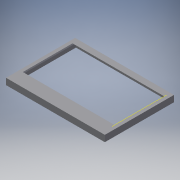
# Autodesk Inventor part: Auschnitt2
Saved by Autodesk Inventor 2017 SP1 (Build 210196100, 196)
## iProperties
Part Number: Auschnitt2
Material: Generisch
Document SubType Name: Modeling
Designer: aXe
Density: 1 g/cm^3
Appearance: Vorgabe
Author: aXe
Autodesk Inventor part; units mm, degrees
ref_plane "YZ Plane" through (0, 0, 0) normal (1, 0, 0) x (0, 1, 0)
ref_plane "Arbeitsebene1" through (47.05, -25.35, -1.6) normal (1, 0, 0) x (0, 1, 0)
sketch "Skizze1" plane through (47.05, -25.35, -1.6) normal (1, 0, 0) x (0, 1, 0)
  line L0 (0, 0) -> (50.7, 0) projected
  line L1 (50.7, 0) -> (50.7, 1.5) projected
  line L2 (0, 1.5) -> (50.7, 1.5) projected
  line L3 (0, 0) -> (0, 1.5) projected
  line L4 (-10, -1.15) -> (53.1, -1.15) projected
  line L5 (53.1, -1.15) -> (53.1, 0) projected
  line L6 (-10, 0) -> (53.1, 0) projected
  line L7 (-10, -1.15) -> (-10, 0) projected
  line L8 (0, 1.5) -> (-0.15, 1.5)
  line L9 (50.7, 1.5) -> (50.85, 1.5)
  line L10 (50.85, 1.5) -> (50.85, 1.3)
  line L11 (53.1, 0) -> (53.4, 0)
  line L12 (50.85, 1.3) -> (53.4, 0)
  line L13 (58.1558, 1.5) -> (50.85, 1.5)
  line L14 (-0.15, 1.5) -> (-0.15, 1.3)
  line L15 (-10, 0) -> (-10.3, 0)
  line L16 (-10, -1.15) -> (-18.8032, -1.15)
  line L17 (-0.15, 1.3) -> (-10.3, 0)
  line L18 (53.4, 0) -> (54.4, -1)
  line L19 (54.4, -1) -> (54.55, -1.15)
  line L20 (54.55, -1.15) -> (55.55, -1.15)
  line L21 (55.55, -1.15) -> (57.05, -1.15)
  line L22 (57.05, -1.15) -> (57.05, 1.5)
  line L23 (-10.3, 0) -> (-11.45, -1.15)
  line L24 (-11.45, -1.15) -> (-13.95, -1.15)
  line L25 (-13.95, -1.15) -> (-13.95, 1.5)
  line L26 (-13.95, 1.5) -> (-0.15, 1.5)
  point P0 (25.35, 1.6)
  dimension "d0" = 0.15
  dimension "d1" = 0.15
  dimension "d2" = 0.2
  dimension "d3" = 0.3
  dimension "d5" = 0.2
  dimension "d6" = 0.3
  dimension "d9" = 1
  dimension "d10" = 1.5
  dimension "d11" = 2.5
  constraints: 38 end point, 6 horizontal, 4 point on line, 3 perpendicular, 1 parallel, 1 vertical
  measures "d0" distance of L2.start L8.end
  measures "d1" distance of L1.end L9.end
  measures "d2" distance of L9.end L10.end
  measures "d3" distance of L5.end L11.end
  measures "d5" distance of L8.end L14.end
  measures "d6" distance of L6.start L15.end
  measures "d9" distance of L19.end L20.end
  measures "d10" distance of L20.end L21.end
  measures "d11" distance of L23.end L24.end
ref_plane "Arbeitsebene2" through (-47.05, -25.35, -1.6) normal (-1, 0, 0) x (0, 0, 1)
extrude "Extrusion1" add sketch "Skizze1" against normal up to surface (94.1 mm away) contours L14 L17 L23 L16 L25 L26 | L13 L22 L21 L20 L19 L18 L12 L10
sketch "Skizze2" plane through (47.05, 31.7, -0.1) normal (0, 1, 0) x (1, 0, 0)
  line L0 (0, 1.5) -> (-94.1, 1.5) projected
  line L1 (-94.1, 1.5) -> (-94.1, 0) projected
  line L2 (0, 0) -> (-94.1, 0) projected
  line L3 (0, 1.5) -> (0, 0) projected
  line L4 (0, 2.65) -> (-94.1, 2.65) projected
  line L5 (-94.1, 2.65) -> (-94.1, 1.5) projected
  line L6 (0, 1.5) -> (-94.1, 1.5) projected
  line L7 (0, 2.65) -> (0, 1.5) projected
  line L8 (0, 0) -> (-94.1, 0) projected
  line L9 (-94.1, 0) -> (-94.3, 0)
  line L10 (-94.3, 0) -> (-95.3, 0)
  line L11 (0, 2.65) -> (-94.1, 2.65) projected
  line L12 (-94.1, 2.65) -> (-95.3, 2.65)
  line L13 (-95.3, 2.65) -> (-94.3, 0)
  line L14 (-95.3, 2.65) -> (-97.8, 2.65)
  line L15 (-97.8, 2.65) -> (-97.8, 0)
  line L16 (-97.8, 0) -> (-95.3, 0)
  line L17 (0, 0) -> (0.2, 0)
  line L18 (0.2, 0) -> (0, 2.65)
  line L19 (0, 2.65) -> (1.2, 2.65)
  line L20 (1.2, 2.65) -> (0.2, 0)
  line L21 (1.2, 2.65) -> (3.7, 2.65)
  line L22 (3.7, 2.65) -> (3.7, 0)
  line L23 (0.2, 0) -> (3.7, 0)
  point P0 (-47.05, -0.1)
  dimension "d14" = 0.2
  dimension "d15" = 1
  dimension "d16" = 1.2
  dimension "d17" = 2.5
  dimension "d18" = 0.2
  dimension "d19" = 1.2
  dimension "d20" = 2.5
  constraints: 28 end point, 5 point on line, 4 perpendicular, 2 horizontal, 1 parallel
  measures "d14" distance of L1.end L9.end
  measures "d15" distance of L9.end L10.end
  measures "d16" distance of L4.end L12.end
  measures "d17" distance of L12.end L14.end
  measures "d18" distance of L2.start L17.end
  measures "d19" distance of L4.start L19.end
  measures "d20" distance of L19.end L21.end
extrude "Extrusion2" add sketch "Skizze2" against normal up to surface (71 mm away) contours L20 L21 L22 L23 | L10 L16 L15 L14 L13
sketch "Skizze3" plane through (-47.05, -39.3, -0.1) normal (-1, 0, 0) x (0, 0, 1)
  line L0 (0, 0) -> (-2.65, 0) projected
  line L1 (0, 13.8) -> (0, 0) projected
  line L2 (-0.2, 13.8) -> (0, 13.8) projected
  line L3 (-1.5, 3.65) -> (-0.2, 13.8) projected
  line L4 (-2.65, 2.5) -> (-1.5, 3.65) projected
  line L5 (-2.65, 0) -> (-2.65, 2.5) projected
  line L6 (-2.65, 68.5) -> (-2.65, 71) projected
  line L7 (-1.5, 67.35) -> (-2.65, 68.5) projected
  line L8 (-0.2, 64.8) -> (-1.5, 67.35) projected
  line L9 (0, 64.8) -> (-0.2, 64.8) projected
  line L10 (0, 71) -> (0, 64.8) projected
  line L11 (-2.65, 71) -> (0, 71) projected
  point P0 (0.1, 39.3)
extrude "Extrusion3" add sketch "Skizze3" along normal up to surface (3.7 mm away)
sketch "Skizze4" plane through (47.05, -25.35, -1.6) normal (1, 0, 0) x (0, 0, -1)
  line L0 (-1.5, -0.15) -> (-1.5, -13.95) projected
  line L1 (-1.5, -13.95) -> (1.15, -13.95) projected
  line L2 (1.15, -13.95) -> (1.15, -11.45) projected
  line L3 (1.15, -11.45) -> (0, -10.3) projected
  line L4 (0, -10.3) -> (-1.3, -0.15) projected
  line L5 (-1.3, -0.15) -> (-1.5, -0.15) projected
  line L6 (0, 53.4) -> (1.15, 54.55) projected
  line L7 (1.15, 54.55) -> (1.15, 57.05) projected
  line L8 (1.15, 57.05) -> (-1.5, 57.05) projected
  line L9 (-1.5, 57.05) -> (-1.5, 50.85) projected
  line L10 (-1.5, 50.85) -> (-1.3, 50.85) projected
  line L11 (-1.3, 50.85) -> (0, 53.4) projected
  point P0 (-1.6, 25.35)
extrude "Extrusion4" add sketch "Skizze4" along normal up to surface (3.7 mm away)
sketch "Skizze5" plane through (50.75, 31.7, -2.75) normal (0, 0, -1) x (-1, 0, 0)
  line L0 (97.8, -69) -> (3.7, -69) projected
  line L1 (97.8, -2) -> (97.8, -69) projected
  line L2 (3.7, -2) -> (97.8, -2) projected
  line L3 (3.7, -69) -> (3.7, -2) projected
  line L4 (2.5, -2.5) -> (2.5, -68.5) projected
  line L5 (99, -2.5) -> (99, -68.5) projected
  line L6 (99, -2.5) -> (2.5, -2.5) projected
  line L7 (99, -68.5) -> (2.5, -68.5) projected
  line L8 (3.7, -2) -> (3.7, -1.7)
  line L9 (3.7, -1.7) -> (2.5, -2.5)
  line L10 (2.5, -2.5) -> (2.5, -1.7)
  line L11 (97.8, -69) -> (97.8, -69.3)
  line L12 (0, -71) -> (101.5, -71) projected
  line L13 (97.8, -69.3) -> (99, -68.5)
  line L14 (99, -68.5) -> (99, -69.3)
  line L15 (0, 0) -> (101.5, 0) projected
  line L16 (0, 0) -> (0, -71) projected
  line L17 (0, -71) -> (101.5, -71) projected
  line L18 (101.5, 0) -> (101.5, -71) projected
  line L19 (99, -2.5) -> (2.5, -2.5) projected
  line L20 (99, -2.5) -> (99, -68.5) projected
  line L21 (99, -68.5) -> (2.5, -68.5) projected
  line L22 (2.5, -2.5) -> (2.5, -68.5) projected
  line L23 (2.5, -1.7) -> (99, -1.7)
  line L24 (99, -1.7) -> (99, -69.3)
  line L25 (99, -69.3) -> (2.5, -69.3)
  line L26 (2.5, -69.3) -> (2.5, -1.7)
  point P0 (50.75, -31.7)
  dimension "d27" = 0.3
  dimension "d28" = 0.3
  constraints: 20 end point, 3 vertical, 2 parallel, 2 perpendicular, 1 horizontal
  measures "d27" distance of L2.start L8.end
  measures "d28" distance of L0.start L11.end
ref_plane "Arbeitsebene3" through (-47.05, -37.3, -6.6) normal (0, 0, -1) x (0, 1, 0)
extrude "Extrusion5" add sketch "Skizze5" along normal up to surface (3.85 mm away)
